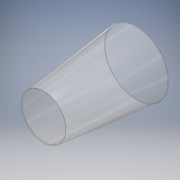
# Autodesk Inventor part: Topf
Saved by Autodesk Inventor 2017.3 (Build 213257000, 257)
## iProperties
Created: 2020-01-20
Part Number: Topf
Material: PET Plastic
Document SubType Name: Modeling
Designer: Ole Simmering
Density: 1.541 g/cm^3
Appearance: Polycarbonate - Clear
Author: Ole Simmering
Autodesk Inventor part; units mm, degrees
ref_plane "YZ Plane" through (0, 0, 0) normal (1, 0, 0) x (0, 1, 0)
ref_plane "XY Plane" through (0, 0, 0) normal (0, 0, 1) x (1, 0, 0)
sketch "Sketch1" plane through (0, 0, 0) normal (0, 1, 0) x (-1, 0, 0)
  circle A0 centre (0, 0) radius 87.5
  dimension "d0" = 175
  constraints: 1 centre point, 1 coincident
  measures "d0" diameter of A0
ref_plane "Work Plane1" through (0, 363, 0) normal (0, 1, 0) x (-1, 0, 0)
sketch "Sketch2" plane through (0, 363, 0) normal (0, 1, 0) x (-1, 0, 0)
  circle A0 centre (0, 0) radius 125
  dimension "d2" = 250
  constraints: 1 centre point, 1 coincident
  measures "d2" diameter of A0
loft "Loft1" add profiles "Sketch1", "Sketch2"
shell "Shell1" thickness 2.5 removed faces 1 at (0.6944, 363, 22.8612)
body "Solid1"
